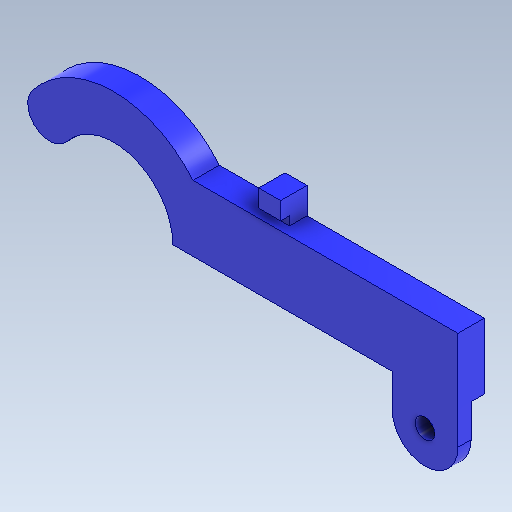
# Autodesk Inventor part: エアタンクペットボトル抑え２
Saved by Autodesk Inventor 2021.3 (Build 253353010, 353A)
## iProperties
Created: 2020-02-08
Part Number: エアタンクペットボトル抑え２
Material: 一般
Document SubType Name: Modeling
Designer: yuta2
Density: 1 g/cm^3
Appearance: 青 - 壁塗料 - 光沢
Author: yuta2
Autodesk Inventor part; units mm, degrees
ref_plane "YZ Plane" through (0, 0, 0) normal (1, 0, 0) x (0, 1, 0)
ref_plane "XZ Plane" through (0, 0, 0) normal (0, 1, 0) x (-1, 0, 0)
ref_plane "XY Plane" through (0, 0, 0) normal (0, 0, 1) x (1, 0, 0)
sketch "スケッチ4" plane through (0, 0, 0) normal (0, 0, 1) x (1, 0, 0)
  circle A0 centre (0, 0) radius 13.5
  circle A1 centre (0, 0) radius 23.5
  circle A2 centre (-14.5779, 11.3901) radius 5
  line L0 (13.5, 0) -> (78.5, 0)
  line L1 (78.5, 0) -> (78.5, 15)
  line L2 (78.5, 15) -> (13.5, 15)
  line L3 (13.5, 15) -> (13.5, 0)
  circle A3 centre (71, -7.5) radius 7.5
  line L4 (63.5, 0) -> (78.5, 0)
  line L5 (78.5, 0) -> (78.5, -7.5)
  line L6 (78.5, -7.5) -> (63.5, -7.5)
  line L7 (63.5, -7.5) -> (63.5, 0)
  point P0 (-10.6379, 8.3117)
  point P1 (78.5, 0)
  point P2 (18.0901, 15)
  point P3 (-18.5179, 14.4685)
  dimension "d15" = 27
  dimension "d19" = 15
  dimension "d16" = 47
  dimension "d17" = 65
  dimension "d18" = 15
  constraints: 16 end point, 4 parallel, 3 horizontal, 2 centre point, 2 coincident, 2 perpendicular, 1 point on line, 1 tangent, 1 vertical, 7 other
  measures "d16" diameter of A1
  measures "d17" distance of L2.end L1.end
  measures "d18" distance of L1.end L0.end
extrude "押し出し3" add sketch "スケッチ4" along normal blind 6 contours L3 L2 A1 L0 | A0 A2 A1 L2 L3 | A2 | A1 L2 L1 L0 | L0 A3 L7 | L0 L5 A3 | A3 L6 | L6 A3
sketch "スケッチ5" plane through (0, 0, 0) normal (0, 0, -1) x (-1, 0, 0)
  line L0 (-78.5, -7.5) -> (-78.5, 15) projected
  line L1 (-63.5, 0) -> (-63.5, -7.5) projected
  line L2 (-78.5, 0) -> (-63.5, 0)
  line L3 (-63.5, 0) -> (-63.5, -7.5)
  line L4 (-63.5, -7.5) -> (-78.5, -7.5)
  line L5 (-78.5, -7.5) -> (-78.5, 0)
  circle A0 centre (-71, -7.5) radius 7.5
  point P0 (0, 0)
  constraints: 8 end point, 2 parallel, 1 horizontal, 1 midpoint, 1 perpendicular, 1 point on line, 3 other
extrude "押し出し4" cut sketch "スケッチ5" against normal blind 3
sketch "スケッチ6" plane through (0, 0, 3) normal (0, 0, -1) x (-1, 0, 0)
  arc A0 (-78.5, -7.5) -> (-63.5, -7.5) centre (-71, -7.5) ccw projected
  point P0 (0, 0)
  constraints: 1 coincident
hole "穴2" at (71, -7.5, 3) direction (0, 0, 1) diameter 4.5 end through all
sketch "スケッチ7" plane through (18.0901, 15, 0) normal (0, 1, 0) x (1, 0, 0)
  line L0 (60.4099, -6) -> (0, -6) projected
  line L1 (-4.5901, 0) -> (60.4099, 0) projected
  line L2 (15, -6) -> (20, -6)
  line L3 (20, -6) -> (20, 0)
  line L4 (20, 0) -> (15, 0)
  line L5 (15, 0) -> (15, -6)
  line L6 (0, 0) -> (0, -6) projected
  point P0 (-18.0901, 0)
  dimension "d31" = 5
  dimension "d32" = 15
  constraints: 8 end point, 2 parallel, 2 point on line, 1 horizontal, 1 perpendicular
  measures "d31" distance of L4.end L3.end
  measures "d32" distance between parallel lines of L5 L6
extrude "押し出し5" add sketch "スケッチ7" along normal blind 6 contours L0 L5 L1 L3
sketch "スケッチ8" plane through (38.0901, 15, 6) normal (1, 0, 0) x (0, 0, -1)
  line L0 (0, 0) -> (2, 0)
  line L1 (2, 0) -> (2, 2)
  line L2 (2, 2) -> (0, 2)
  line L3 (0, 2) -> (0, 0)
  point P0 (6, -15)
  dimension "d35" = 2
  dimension "d36" = 2
  constraints: 8 end point, 2 parallel, 1 horizontal, 1 perpendicular
  measures "d35" distance of L2.end L1.end
  measures "d36" distance of L1.end L0.end
extrude "押し出し6" cut sketch "スケッチ8" against normal blind 6
